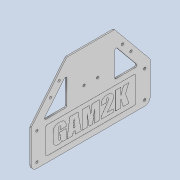
# Autodesk Inventor part: X Axis V Wheel Outside Frame Machined
Saved by Autodesk Inventor 2022 (Build 260153000, 153)
## iProperties
Created: 2021-10-10
Part Number: X Axis V Wheel Outside Frame Machined
Material: Generic
Document SubType Name: Modeling
Designer: Coy
Density: 1 g/cm^3
Appearance: Machined - Aluminum
Author: Coy
Autodesk Inventor part; units mm, degrees
ref_plane "YZ Plane" through (0, 0, 0) normal (1, 0, 0) x (0, 1, 0)
ref_plane "XZ Plane" through (0, 0, 0) normal (0, 1, 0) x (-1, 0, 0)
ref_plane "XY Plane" through (0, 0, 0) normal (0, 0, 1) x (1, 0, 0)
sketch "Sketch1" plane through (0, 0, 0) normal (1, 0, 0) x (0, 1, 0)
  line L0 (0.014, 0) -> (40.014, 0) construction
  line L1 (40.014, 0) -> (40.014, 66.5) construction
  line L2 (40.014, 66.5) -> (0.014, 66.5) construction
  line L3 (0.014, 66.5) -> (0.014, 0) construction
  line L4 (0.014, 66.5) -> (40.014, 66.5) construction
  line L5 (40.014, 66.5) -> (40.014, 86.5) construction
  line L6 (40.014, 86.5) -> (0.014, 86.5) construction
  line L7 (0.014, 86.5) -> (0.014, 66.5) construction
  line L8 (0.014, 0) -> (40.014, 0) construction
  line L9 (40.014, 0) -> (40.014, -20) construction
  line L10 (40.014, -20) -> (0.014, -20) construction
  line L11 (0.014, -20) -> (0.014, 0) construction
  line L12 (48.214, 61.45) -> (-8.186, 61.45) construction
  line L13 (-8.186, 61.45) -> (-8.186, 5.05) construction
  line L14 (-8.186, 5.05) -> (48.214, 5.05) construction
  line L15 (48.214, 5.05) -> (48.214, 61.45) construction
  line L16 (48.214, 33.25) -> (-8.186, 33.25) construction
  line L17 (40.014, 33.25) -> (0.014, 33.25) construction
  line L18 (43.584, 56.82) -> (-3.556, 56.82) construction
  line L19 (-3.556, 56.82) -> (-3.556, 9.68) construction
  line L20 (-3.556, 9.68) -> (43.584, 9.68) construction
  line L21 (43.584, 9.68) -> (43.584, 56.82) construction
  line L22 (43.584, 56.82) -> (48.214, 56.82) construction
  line L23 (43.584, 56.82) -> (43.584, 61.45) construction
  line L24 (-3.556, 9.68) -> (-8.186, 9.68) construction
  line L25 (-3.556, 9.68) -> (-3.556, 5.05) construction
  line L26 (40.014, -10) -> (0.014, -10) construction
  line L27 (40.014, 76.5) -> (0.014, 76.5) construction
  circle A0 centre (30.014, 76.5) radius 2.1
  circle A1 centre (10.014, 76.5) radius 2.1
  circle A2 centre (30.014, -10) radius 2.1
  circle A3 centre (10.014, -10) radius 2.1
  circle A4 centre (43.584, 56.82) radius 2.6
  circle A5 centre (43.584, 9.68) radius 2.6
  circle A6 centre (-3.556, 9.68) radius 2.6
  circle A7 centre (-3.556, 56.82) radius 2.6
  circle A8 centre (20.014, 33.25) radius 19.15
  circle A9 centre (-24.986, 18.25) radius 11.08 construction
  circle A10 centre (-24.986, 18.25) radius 13 construction
  circle A11 centre (-24.986, 18.25) radius 2.5
  line L28 (-59.986, 153.25) -> (-59.986, -86.75) construction
  circle A12 centre (-59.986, -86.75) radius 2.6
  circle A13 centre (-59.986, 153.25) radius 2.6
  line L29 (-120.432, 153.25) -> (-120.432, -86.75) construction
  circle A14 centre (-120.432, -86.75) radius 2.6
  circle A15 centre (-120.432, 153.25) radius 2.6
  circle A16 centre (-59.986, -86.75) radius 12 construction
  circle A17 centre (-120.432, -86.75) radius 12 construction
  circle A18 centre (-120.432, 153.25) radius 12 construction
  circle A19 centre (-59.986, 153.25) radius 12 construction
  line L30 (-110, 482.7599) -> (-70, 482.7599) construction
  line L31 (-70, -517.2401) -> (-110, -517.2401) construction
  circle A20 centre (-24.986, 48.25) radius 2.5
  circle A21 centre (-24.986, 48.25) radius 11.08 construction
  circle A22 centre (-24.986, 48.25) radius 13 construction
  circle A23 centre (20.014, 33.25) radius 11.08 construction
  circle A24 centre (20.014, 33.25) radius 13 construction
  line L32 (-23.1733, 29.1807) -> (18.2013, 22.3193) construction
  line L33 (18.2013, 44.1807) -> (-23.1733, 37.3193) construction
  line L34 (-120.8194, -99.25) -> (-47.8194, -99.25)
  line L35 (-47.8194, 165.75) -> (-120.8194, 165.75)
  line L36 (-132.8194, 153.75) -> (-132.8194, -87.25)
  line L37 (-59.986, 153.25) -> (-120.432, 153.25) construction
  line L38 (-120.432, -86.75) -> (-59.986, -86.75) construction
  line L39 (-59.986, 153.25) -> (-59.986, 165.75) construction
  line L40 (-120.432, -86.75) -> (-120.432, -99.25) construction
  line L41 (48.3416, -20) -> (48.3416, 86.5)
  line L42 (-47.8194, 165.75) -> (48.3416, 86.5)
  line L43 (17.6122, 86.5) -> (40.014, 86.5) construction
  arc A25 (-120.8194, 165.75) -> (-132.8194, 153.75) centre (-120.8194, 153.75) ccw
  arc A26 (-132.8194, -87.25) -> (-120.8194, -99.25) centre (-120.8194, -87.25) ccw
  line L44 (48.3416, -20) -> (-47.8194, -99.25)
  line L45 (-47.8194, 165.75) -> (-47.8194, -99.25) construction
  line L46 (-120.432, -86.75) -> (-132.8194, -86.75) construction
  line L47 (-59.986, 153.25) -> (-47.8194, 153.25) construction
  line L48 (-36.066, 48.25) -> (-36.066, 286.613) construction
  line L49 (-47.8194, 139.8332) -> (16.8944, 86.5)
  line L50 (-47.8194, 139.8332) -> (-47.8194, 86.5)
  line L51 (-47.8194, 86.5) -> (16.8944, 86.5)
  line L52 (-47.8194, -73.3332) -> (16.8944, -20)
  line L53 (-47.8194, -20) -> (16.8944, -20)
  line L54 (-47.8194, -73.3332) -> (-47.8194, -20)
  point P0 (-132.8194, -99.25)
  point P1 (-132.8194, 165.75)
  dimension "d122" = 22.16
  dimension "d97" = 40
  dimension "d98" = 66.5
  dimension "d99" = 40
  dimension "d100" = 20
  dimension "d101" = 40
  dimension "d102" = 20
  dimension "d103" = 56.4
  dimension "d104" = 56.4
  dimension "d105" = 0
  dimension "d106" = 8.2
  dimension "d107" = 47.14
  dimension "d108" = 47.14
  dimension "d109" = 4.2
  dimension "d110" = 20
  dimension "d111" = 10
  dimension "d112" = 10
  dimension "d113" = 20
  dimension "d114" = 4.2
  dimension "d115" = 4.2
  dimension "d116" = 4.2
  dimension "d117" = 5.2
  dimension "d118" = 5.2
  dimension "d119" = 5.2
  dimension "d120" = 5.2
  dimension "d121" = 38.3
  dimension "d123" = 26
  dimension "d124" = 5
  dimension "d125" = 240
  dimension "d126" = 60
  dimension "d127" = 5.2
  dimension "d128" = 5.2
  dimension "d129" = 5.2
  dimension "d130" = 5.2
  dimension "d131" = 60.446
  dimension "d132" = 24
  dimension "d133" = 24
  dimension "d134" = 24
  dimension "d135" = 24
  dimension "d136" = 40
  dimension "d137" = 1000
  dimension "d138" = 45
  dimension "d139" = 5
  dimension "d140" = 22.16
  dimension "d141" = 26
  dimension "d142" = 45
  dimension "d143" = 22.16
  dimension "d144" = 26
  dimension "d145" = 15
  dimension "d146" = 15
  dimension "d147" = 265
  dimension "d148" = 85
  dimension "d149" = 106.5
  dimension "d150" = 12
  dimension "d151" = 72.8333
  dimension "d152" = 28.3276
  dimension "d153" = 53.25
  dimension "d154" = 85
  dimension "d155" = 132.5
  dimension "d156" = 60.446
  dimension "d157" = 20
  constraints: 110 end point, 26 centre point, 20 point on line, 18 coincident, 17 parallel, 14 perpendicular, 9 midpoint, 8 horizontal, 8 point on circle, 8 tangent, 4 vertical, 3 symmetric about line, 1 equal radius, 4 other
  measures "d97" distance of L2.end L1.end
  measures "d98" distance of L1.end L0.end
  measures "d99" distance of L5.end L6.end
  measures "d100" distance of L5.end L4.end
  measures "d101" distance of L9.end L10.end
  measures "d102" distance of L9.end L8.end
  measures "d103" distance of L14.end L13.end
  measures "d104" distance of L13.end L12.end
  measures "d105" distance between parallel lines of L17 L16
  measures "d106" distance between parallel lines of L15 L1
  measures "d107" distance of L20.end L18.start
  measures "d108" distance of L19.end L20.end
  measures "d109" diameter of A0
  measures "d110" distance of A1.centre A0.centre
  measures "d111" distance from line of L5 A0.centre
  measures "d112" distance from line of L9 A2.centre
  measures "d113" distance of A2.centre A3.centre
  measures "d114" diameter of A1
  measures "d115" diameter of A2
  measures "d116" diameter of A3
  measures "d117" diameter of A4
  measures "d118" diameter of A5
  measures "d119" diameter of A6
  measures "d120" diameter of A7
  measures "d121" diameter of A8
  measures "d123" diameter of A10
  measures "d124" diameter of A11
  measures "d125" distance of L28.start L28.end
  measures "d126" distance between parallel lines of L7 L28
  measures "d127" diameter of A12
  measures "d128" diameter of A13
  measures "d129" diameter of A14
  measures "d130" diameter of A15
  measures "d131" distance between parallel lines of L28 L29
  measures "d132" diameter of A16
  measures "d133" diameter of A17
  measures "d134" diameter of A18
  measures "d135" diameter of A19
  measures "d136" distance of L31.start L31.end
  measures "d137" distance of L30.end L31.start
  measures "d138" horizontal distance of A8.centre point (-24.986, 18.25)
  measures "d139" diameter of A20
  measures "d140" diameter of A21
  measures "d141" diameter of A22
  measures "d142" horizontal distance of A8.centre A20.centre
  measures "d143" diameter of A23
  measures "d144" diameter of A24
  measures "d145" vertical distance of A8.centre A10.centre
  measures "d146" vertical distance of A23.centre A21.centre
  measures "d147" distance of point (-132.819, 165.75) point (-132.819, -99.25)
  measures "d148" distance of L35.start point (-132.819, 165.75)
  measures "d149" distance of L41.end L41.start
  measures "d150" radius of A25
  measures "d151" distance between parallel lines of L28 L36
  measures "d152" distance from line of A8.centre L41
  measures "d153" vertical distance of L41.end A23.centre
  measures "d154" distance of L34.end point (-132.819, -99.25)
  measures "d155" vertical distance of L35.start A24.centre
  measures "d156" distance of L37.start L37.end
  measures "d157" distance between parallel lines of L42 L49
extrude "Extrusion1" add sketch "Sketch1" along normal blind 3.175 contours A0 | A1 | A2 | A3 | A4 | A5 | A6 | A7 | A8 | A26 L36 A25 L35 L42 L41 L44 L34
sketch "Sketch4" plane through (3.175, 0, 0) normal (1, 0, 0) x (0, 0, -1)
  line L0 (-130.075, -59.986) -> (63.575, -59.986)
  line L1 (66.75, -63.161) -> (66.75, -116.811)
  line L2 (63.575, -119.986) -> (-130.075, -119.986)
  line L3 (-133.25, -116.811) -> (-133.25, -63.161)
  arc A0 (-130.075, -59.986) -> (-133.25, -63.161) centre (-130.075, -63.161) ccw
  arc A1 (-133.25, -116.811) -> (-130.075, -119.986) centre (-130.075, -116.811) ccw
  arc A2 (63.575, -119.986) -> (66.75, -116.811) centre (63.575, -116.811) ccw
  arc A3 (66.75, -63.161) -> (63.575, -59.986) centre (63.575, -63.161) ccw
  circle A4 centre (-153.25, -59.986) radius 2.6 projected
  point P0 (0, 0)
  point P1 (-133.25, -59.986)
  point P2 (66.75, -59.986)
  point P3 (-133.25, -119.986)
  dimension "d82" = 200
  dimension "d83" = 60
  dimension "d84" = 0
  dimension "d85" = 20
  dimension "d86" = 3.175
  dimension "d158" = 0
  dimension "d159" = 0
  constraints: 8 end point, 8 point on circle, 8 tangent, 6 point on line, 4 centre point, 3 equal radius, 2 parallel, 1 horizontal, 1 perpendicular
  measures "d82" distance of point (-133.25, -59.986) point (66.75, -59.986)
  measures "d83" distance of point (-133.25, -119.986) point (-133.25, -59.986)
  measures "d84" distance from line of point (-153.25, -59.986) L0
  measures "d85" distance from line of L3 point (-153.25, -59.986)
  measures "d86" radius of A0
  measures "d158" distance of A4.centre point (-153.25, -59.986)
  measures "d159" distance of A4.centre point (-153.25, -59.986)
extrude "Extrusion4" cut sketch "Sketch4" against normal blind 0.127 contours L0 A3 L1 A2 L2 A1 L3 A0
sketch "Sketch5" plane through (3.048, 0, 0) normal (1, 0, 0) x (0, 0, -1)
  line L0 (-133.8465, -59.4324) -> (66.5544, -59.4324) construction
  line L1 (66.5544, -59.4324) -> (66.5544, -120.155) construction
  line L2 (66.5544, -120.155) -> (-133.8465, -120.155) construction
  line L3 (-133.8465, -120.155) -> (-133.8465, -59.4324) construction
  line L4 (-87.9791, -84.5036) -> (-100.4584, -84.5036)
  line L5 (-100.4584, -84.5036) -> (-100.4584, -80.8864)
  spline S0 degree 2 poles (-100.4584, -80.8864) (-100.4584, -77.4501) (-101.1517, -75.7319) (-102.478, -75.7319) knots 0 0 0 1 2 2 2
  spline S1 degree 2 poles (-102.478, -75.7319) (-103.6536, -75.7319) (-104.4675, -77.209) (-104.4675, -80.2836) knots 0 0 0 1 2 2 2
  line L6 (-104.4675, -80.2836) -> (-104.4675, -99.4546)
  spline S2 degree 2 poles (-104.4675, -99.4546) (-104.4675, -102.1374) (-103.6536, -103.8555) (-102.3876, -103.8555) knots 0 0 0 1 2 2 2
  spline S3 degree 2 poles (-102.3876, -103.8555) (-101.0311, -103.8555) (-100.0665, -101.9264) (-100.0665, -99.123) knots 0 0 0 1 2 2 2
  line L7 (-100.0665, -99.123) -> (-100.0665, -94.3906)
  line L8 (-100.0665, -94.3906) -> (-102.5684, -94.3906)
  line L9 (-102.5684, -94.3906) -> (-102.5684, -88.3016)
  line L10 (-102.5684, -88.3016) -> (-87.9791, -88.3016)
  line L11 (-87.9791, -88.3016) -> (-87.9791, -109.7937)
  line L12 (-87.9791, -109.7937) -> (-95.8164, -109.7937)
  line L13 (-95.8164, -109.7937) -> (-96.9618, -106.9301)
  spline S4 degree 2 poles (-96.9618, -106.9301) (-98.258, -108.7689) (-102.1464, -110.6377) (-104.7689, -110.6377) knots 0 0 0 1 2 2 2
  spline S5 degree 2 poles (-104.7689, -110.6377) (-107.9038, -110.6377) (-113.3898, -108.1057) (-116.2233, -104.3378) (-116.9467, -100.2082) (-116.9467, -96.0786) knots 0 0 0 1 2 3 4 4 4
  line L14 (-116.9467, -96.0786) -> (-116.9467, -84.2022)
  spline S6 degree 2 poles (-116.9467, -84.2022) (-116.9467, -78.475) (-115.4697, -73.2602) (-108.4464, -68.9497) (-102.8699, -68.9497) knots 0 0 0 1 2 3 3 3
  spline S7 degree 2 poles (-102.8699, -68.9497) (-97.3838, -68.9497) (-90.1796, -72.6875) (-87.9791, -77.8721) (-87.9791, -82.7854) knots 0 0 0 1 2 3 3 3
  line L15 (-87.9791, -82.7854) -> (-87.9791, -84.5036)
  line L16 (-61.5737, -69.7937) -> (-54.4298, -109.7937)
  line L17 (-54.4298, -109.7937) -> (-67.2105, -109.7937)
  line L18 (-67.2105, -109.7937) -> (-67.8736, -102.5895)
  line L19 (-67.8736, -102.5895) -> (-72.3348, -102.5895)
  line L20 (-72.3348, -102.5895) -> (-73.0583, -109.7937)
  line L21 (-73.0583, -109.7937) -> (-85.9595, -109.7937)
  line L22 (-85.9595, -109.7937) -> (-79.6295, -69.7937)
  line L23 (-79.6295, -69.7937) -> (-61.5737, -69.7937)
  spline S8 degree 2 poles (-68.1751, -95.5059) (-69.1095, -88.7236) (-70.0741, -78.7161) knots 0 0 0 1 1 1
  spline S9 degree 2 poles (-70.0741, -78.7161) (-71.9731, -90.2007) (-72.4554, -95.5059) knots 0 0 0 1 1 1
  line L24 (-72.4554, -95.5059) -> (-68.1751, -95.5059)
  line L25 (-13.7968, -69.7937) -> (-13.7968, -109.7937)
  line L26 (-13.7968, -109.7937) -> (-24.7086, -109.7937)
  line L27 (-24.7086, -109.7937) -> (-24.7086, -82.7854)
  line L28 (-24.7086, -82.7854) -> (-29.0794, -109.7937)
  line L29 (-29.0794, -109.7937) -> (-36.796, -109.7937)
  line L30 (-36.796, -109.7937) -> (-41.3476, -83.3883)
  line L31 (-41.3476, -83.3883) -> (-41.3778, -109.7937)
  line L32 (-41.3778, -109.7937) -> (-52.2896, -109.7937)
  line L33 (-52.2896, -109.7937) -> (-52.2896, -69.7937)
  line L34 (-52.2896, -69.7937) -> (-36.163, -69.7937)
  spline S10 degree 2 poles (-36.163, -69.7937) (-35.4697, -73.4109) (-34.686, -78.2941) knots 0 0 0 1 1 1
  line L35 (-34.686, -78.2941) -> (-32.9075, -88.4825)
  line L36 (-32.9075, -88.4825) -> (-30.0741, -69.7937)
  line L37 (-30.0741, -69.7937) -> (-13.7968, -69.7937)
  line L38 (16.7081, -102.9814) -> (16.7081, -109.7937)
  line L39 (16.7081, -109.7937) -> (-9.6672, -109.7937)
  line L40 (-9.6672, -109.7937) -> (-9.6672, -104.0967)
  spline S11 degree 2 poles (-9.6672, -104.0967) (2.0585, -88.1208) (6.4595, -80.5247) (6.4595, -78.3845) knots 0 0 0 1 2 2 2
  spline S12 degree 2 poles (6.4595, -78.3845) (6.4595, -76.7568) (5.1332, -75.1592) (3.7767, -75.1592) knots 0 0 0 1 2 2 2
  spline S13 degree 2 poles (3.7767, -75.1592) (2.3901, -75.1592) (1.0638, -76.9377) (1.0638, -79.5903) knots 0 0 0 1 2 2 2
  line L41 (1.0638, -79.5903) -> (1.0638, -83.3883)
  line L42 (1.0638, -83.3883) -> (-9.6672, -83.3883)
  line L43 (-9.6672, -83.3883) -> (-9.6672, -81.9414)
  spline S14 degree 2 poles (-9.6672, -81.9414) (-9.6672, -78.5654) (-8.8231, -74.6769) (-5.5677, -70.9392) (-0.3529, -69.01) (3.2944, -69.01) knots 0 0 0 1 2 3 4 4 4
  spline S15 degree 2 poles (3.2944, -69.01) (10.4384, -69.01) (17.7631, -74.9181) (17.7631, -79.4395) knots 0 0 0 1 2 2 2
  spline S16 degree 2 poles (17.7631, -79.4395) (17.7631, -82.8759) (13.6335, -90.5322) (3.5356, -102.9814) knots 0 0 0 1 2 2 2
  line L44 (3.5356, -102.9814) -> (16.7081, -102.9814)
  line L45 (51.4632, -69.7937) -> (44.2891, -87.8495)
  line L46 (44.2891, -87.8495) -> (52.1565, -109.7937)
  line L47 (52.1565, -109.7937) -> (39.2854, -109.7937)
  line L48 (39.2854, -109.7937) -> (34.1912, -92.6423)
  line L49 (34.1912, -92.6423) -> (34.1912, -109.7937)
  line L50 (34.1912, -109.7937) -> (21.7119, -109.7937)
  line L51 (21.7119, -109.7937) -> (21.7119, -69.7937)
  line L52 (21.7119, -69.7937) -> (34.1912, -69.7937)
  line L53 (34.1912, -69.7937) -> (34.1912, -85.3476)
  line L54 (34.1912, -85.3476) -> (39.7677, -69.7937)
  line L55 (39.7677, -69.7937) -> (51.4632, -69.7937)
  point P0 (0, 0)
  constraints: 2 other
extrude "Extrusion5" add sketch "Sketch5" along normal up to surface (0.127 mm away)
sketch "Sketch6" plane through (3.175, 0, 0) normal (1, 0, 0) x (0, 0, -1)
  circle A0 centre (-103.7568, 11.6788) radius 2.6
  circle A1 centre (-122.8364, -11.4722) radius 2.6
  line L0 (-33.25, 48.214) -> (-33.25, -69.4164) construction
  circle A2 centre (37.2568, 11.6788) radius 2.6
  circle A3 centre (56.3364, -11.4722) radius 2.6
  line L1 (-139.8332, -47.8194) -> (-86.5, 16.8944) projected
  line L2 (-86.5, 48.3416) -> (-165.75, -47.8194) projected
  line L3 (-113.2966, 0.1033) -> (-121.0136, 6.4632) construction
  line L4 (-113.2966, 0.1033) -> (-103.7568, 11.6788) construction
  line L5 (-113.2966, 0.1033) -> (-122.8364, -11.4722) construction
  line L6 (-113.2966, 0.1033) -> (-105.5796, -6.2566) construction
  point P0 (0, 0)
  point P1 (0, 0)
  dimension "d93" = 5.2
  dimension "d160" = 15
  dimension "d161" = 15
  dimension "d162" = 53.25
  dimension "d164" = 30
  constraints: 10 end point, 4 centre point, 3 perpendicular, 2 point on line, 2 symmetric about line, 1 vertical, 2 other
  measures "d93" diameter of A0
  measures "d160" distance of L3.start L4.end
  measures "d161" distance of L3.start L5.end
  measures "d162" distance from line of L2.start L0
  measures "d164" distance from line of L1.end L6
extrude "Extrusion6" cut sketch "Sketch6" against normal through all
fillet "Fillet2" radius 3.175 10 edges at (1.5875, -47.8194, -20) (1.5875, -47.8194, -73.3332) (1.5875, 16.8944, -20) (1.5875, -47.8194, 86.5) (1.5875, -47.8194, 139.8332) (1.5875, 16.8944, 86.5) (1.5875, -47.8194, 165.75) (1.5875, 48.3416, 86.5) (1.5875, 48.3416, -20) (1.5875, -47.8194, -99.25)
body "Solid1"
